Autodesk Fusion 360 part; units mm, degrees
(part 3 of 5)
  spline S639 degree 3 poles (-49.8546, -125.9974) (-49.939, -126.4512) (-49.939, -126.3246) (-49.9074, -125.2905) knots 0 0 0 0 1 1 1 1
  spline S640 degree 3 poles (-49.9074, -125.2905) (-49.8441, -123.6338) (-49.6436, -122.7158) (-49.3165, -122.4942) knots 0 0 0 0 1 1 1 1
  spline S641 degree 3 poles (-49.3165, -122.4942) (-48.926, -122.2515) (-48.1663, -121.5339) (-48.1663, -121.4179) knots 0 0 0 0 1 1 1 1
  spline S642 degree 3 poles (-48.1663, -121.4179) (-48.1663, -121.3545) (-48.409, -121.5339) (-48.7044, -121.7977) knots 0 0 0 0 1 1 1 1
  spline S643 degree 3 poles (-48.7044, -121.7977) (-49.1371, -122.1882) (-50.1923, -122.8107) (-50.4244, -122.8107) knots 0 0 0 0 1 1 1 1
  spline S644 degree 3 poles (-50.4244, -122.8107) (-50.4561, -122.8107) (-50.2345, -122.5575) (-49.9285, -122.2515) knots 0 0 0 0 1 1 1 1
  spline S645 degree 3 poles (-49.9285, -122.2515) (-49.633, -121.9349) (-49.327, -121.6184) (-49.2637, -121.5339) knots 0 0 0 0 1 1 1 1
  spline S646 degree 3 poles (-49.2637, -121.5339) (-49.2004, -121.4495) (-48.926, -121.2068) (-48.6622, -120.9852) knots 0 0 0 0 1 1 1 1
  spline S647 degree 3 poles (-48.6622, -120.9852) (-48.1979, -120.6054) (-47.4593, -119.6768) (-47.5543, -119.5818) knots 0 0 0 0 1 1 1 1
  spline S648 degree 3 poles (-47.5543, -119.5818) (-47.5859, -119.5607) (-47.8392, -119.8245) (-48.1241, -120.1727) knots 0 0 0 0 1 1 1 1
  spline S649 degree 3 poles (-48.1241, -120.1727) (-48.8944, -121.1013) (-49.7807, -121.7239) (-50.646, -121.9455) knots 0 0 0 0 1 1 1 1
  spline S650 degree 3 poles (-50.646, -121.9455) (-51.7012, -122.2093) (-51.6907, -122.2304) (-50.7093, -121.2596) knots 0 0 0 0 1 1 1 1
  spline S651 degree 3 poles (-50.7093, -121.2596) (-50.0129, -120.5631) (-49.6963, -120.1516) (-49.4431, -119.6346) knots 0 0 0 0 1 1 1 1
  spline S652 degree 3 poles (-49.4431, -119.6346) (-49.2637, -119.2441) (-49.116, -118.8959) (-49.116, -118.8537) knots 0 0 0 0 1 1 1 1
  spline S653 degree 3 poles (-49.116, -118.8537) (-49.116, -118.8115) (-49.2637, -118.9276) (-49.4536, -119.107) knots 0 0 0 0 1 1 1 1
  spline S654 degree 3 poles (-49.4536, -119.107) (-49.7491, -119.4024) (-50.7199, -119.8562) (-51.0364, -119.8562) knots 0 0 0 0 1 1 1 1
  spline S655 degree 3 poles (-51.0364, -119.8562) (-51.0998, -119.8562) (-50.9626, -119.6873) (-50.7304, -119.4868) knots 0 0 0 0 1 1 1 1
  spline S656 degree 3 poles (-50.7304, -119.4868) (-50.1606, -119.0014) (-49.3587, -117.9779) (-48.8311, -117.0599) knots 0 0 0 0 1 1 1 1
  spline S657 degree 3 poles (-48.8311, -117.0599) (-48.314, -116.163) (-47.5015, -113.8732) (-47.8075, -114.1792) knots 0 0 0 0 1 1 1 1
  spline S658 degree 3 poles (-47.8075, -114.1792) (-47.8392, -114.2214) (-48.0186, -114.6962) (-48.2085, -115.2449) knots 0 0 0 0 1 1 1 1
  spline S659 degree 3 poles (-48.2085, -115.2449) (-48.5145, -116.0996) (-49.1898, -117.5242) (-49.4325, -117.7774) knots 0 0 0 0 1 1 1 1
  spline S660 degree 3 poles (-49.4325, -117.7774) (-49.4642, -117.8196) (-49.3903, -117.5136) (-49.2531, -117.0915) knots 0 0 0 0 1 1 1 1
  spline S661 degree 3 poles (-49.2531, -117.0915) (-48.8944, -116.0047) (-48.8944, -116.0363) (-48.8944, -114.5801) knots 0 0 0 0 1 1 1 1
  spline S662 degree 3 poles (-48.8944, -114.5801) (-48.8838, -111.5412) (-49.8124, -108.5233) (-51.3213, -106.6872) knots 0 0 0 0 1 1 1 1
  spline S663 degree 3 poles (-51.3213, -106.6872) (-51.9334, -105.9591) (-51.8912, -106.1807) (-51.2791, -107.0038) knots 0 0 0 0 1 1 1 1
  spline S664 degree 3 poles (-52.8619, -111.5306) (-52.7142, -111.8261) (-52.6087, -112.0899) (-52.6192, -112.1004) knots 0 0 0 0 1 1 1 1
  spline S665 degree 3 poles (-52.6192, -112.1004) (-52.6403, -112.1215) (-52.8514, -112.1637) (-53.0941, -112.2059) knots 0 0 0 0 1 1 1 1
  line L120 (-53.0941, -112.2059) -> (-53.5373, -112.2798)
  line L121 (-53.5373, -112.2798) -> (-53.5267, -111.0769)
  line L122 (-53.5267, -111.0769) -> (-53.5162, -109.8845)
  line L123 (-53.5162, -109.8845) -> (-53.3262, -110.4332)
  spline S666 degree 3 poles (-53.3262, -110.4332) (-53.2313, -110.7392) (-53.0202, -111.2246) (-52.8619, -111.5306) knots 0 0 0 0 1 1 1 1
  spline S667 degree 3 poles (-59.8263, -110.8553) (-59.8263, -111.0769) (-59.7841, -111.499) (-59.7419, -111.805) knots 0 0 0 0 1 1 1 1
  line L124 (-59.7419, -111.805) -> (-59.668, -112.3537)
  line L125 (-59.668, -112.3537) -> (-60.0584, -112.2481)
  spline S668 degree 3 poles (-60.0584, -112.2481) (-60.7338, -112.0688) (-60.7549, -112.0582) (-60.6388, -111.9105) knots 0 0 0 0 1 1 1 1
  spline S669 degree 3 poles (-60.6388, -111.9105) (-60.5755, -111.8366) (-60.375, -111.4779) (-60.1956, -111.1191) knots 0 0 0 0 1 1 1 1
  spline S670 degree 3 poles (-60.1956, -111.1191) (-60.0162, -110.7603) (-59.8579, -110.4649) (-59.8474, -110.4649) knots 0 0 0 0 1 1 1 1
  spline S671 degree 3 poles (-59.8474, -110.4649) (-59.8368, -110.4649) (-59.8263, -110.6442) (-59.8263, -110.8553) knots 0 0 0 0 1 1 1 1
  spline S672 degree 3 poles (-50.1923, -114.0525) (-49.9812, -114.3691) (-49.6752, -114.8228) (-49.4958, -115.0444) knots 0 0 0 0 1 1 1 1
  spline S673 degree 3 poles (-49.4958, -115.0444) (-49.2215, -115.4032) (-49.2109, -115.4349) (-49.4114, -115.3293) knots 0 0 0 0 1 1 1 1
  spline S674 degree 3 poles (-49.4114, -115.3293) (-50.0551, -114.9811) (-52.4821, -112.2693) (-52.2288, -112.1848) knots 0 0 0 0 1 1 1 1
  spline S675 degree 3 poles (-52.2288, -112.1848) (-52.1655, -112.1637) (-51.9545, -112.0582) (-51.754, -111.9527) knots 0 0 0 0 1 1 1 1
  line L126 (-51.754, -111.9527) -> (-51.3847, -111.7522)
  line L127 (-51.3847, -111.7522) -> (-50.9731, -112.6175)
  spline S676 degree 3 poles (-50.9731, -112.6175) (-50.7515, -113.0818) (-50.4033, -113.736) (-50.1923, -114.0525) knots 0 0 0 0 1 1 1 1
  spline S677 degree 3 poles (-60.0268, -112.4381) (-59.6152, -112.5753) (-59.5836, -112.6175) (-59.4148, -113.2506) knots 0 0 0 0 1 1 1 1
  spline S678 degree 3 poles (-59.4148, -113.2506) (-59.1615, -114.1581) (-58.7816, -114.9495) (-58.3279, -115.5087) knots 0 0 0 0 1 1 1 1
  spline S679 degree 3 poles (-58.3279, -115.5087) (-57.8953, -116.0363) (-57.7897, -116.0258) (-58.0219, -115.4982) knots 0 0 0 0 1 1 1 1
  spline S680 degree 3 poles (-58.0219, -115.4982) (-58.2224, -115.0022) (-58.5495, -113.5249) (-58.4651, -113.4511) knots 0 0 0 0 1 1 1 1
  spline S681 degree 3 poles (-58.4651, -113.4511) (-58.4334, -113.4089) (-58.4018, -113.4511) (-58.4018, -113.5355) knots 0 0 0 0 1 1 1 1
  spline S682 degree 3 poles (-58.4018, -113.5355) (-58.4018, -113.8626) (-57.737, -115.0022) (-57.0722, -115.7936) knots 0 0 0 0 1 1 1 1
  spline S683 degree 3 poles (-57.0722, -115.7936) (-56.5763, -116.3951) (-56.5235, -116.5428) (-56.4918, -117.292) knots 0 0 0 0 1 1 1 1
  spline S684 degree 3 poles (-56.4918, -117.292) (-56.4707, -117.598) (-56.4391, -117.8513) (-56.3969, -117.8513) knots 0 0 0 0 1 1 1 1
  spline S685 degree 3 poles (-56.3969, -117.8513) (-56.3019, -117.8513) (-55.9748, -116.7855) (-55.9748, -116.469) knots 0 0 0 0 1 1 1 1
  spline S686 degree 3 poles (-55.9748, -116.469) (-55.9642, -116.2263) (-55.9537, -116.2368) (-55.7849, -116.5534) knots 0 0 0 0 1 1 1 1
  spline S687 degree 3 poles (-55.7849, -116.5534) (-55.5422, -117.0071) (-54.2865, -118.5899) (-54.1704, -118.5899) knots 0 0 0 0 1 1 1 1
  spline S688 degree 3 poles (-54.1704, -118.5899) (-54.1176, -118.5899) (-54.0649, -118.5055) (-54.0543, -118.4) knots 0 0 0 0 1 1 1 1
  spline S689 degree 3 poles (-54.0543, -118.4) (-54.0438, -118.305) (-54.0332, -118.1467) (-54.0121, -118.0623) knots 0 0 0 0 1 1 1 1
  spline S690 degree 3 poles (-54.0121, -118.0623) (-54.0016, -117.9779) (-53.991, -117.6824) (-53.9805, -117.3975) knots 0 0 0 0 1 1 1 1
  spline S691 degree 3 poles (-53.9805, -117.3975) (-53.9699, -116.9649) (-53.9382, -116.9016) (-53.7483, -116.9016) knots 0 0 0 0 1 1 1 1
  spline S692 degree 3 poles (-53.7483, -116.9016) (-53.5584, -116.9016) (-53.5267, -116.9544) (-53.5689, -117.2076) knots 0 0 0 0 1 1 1 1
  spline S693 degree 3 poles (-53.5689, -117.2076) (-53.6111, -117.482) (-53.5795, -117.5031) (-53.2946, -117.5031) knots 0 0 0 0 1 1 1 1
  spline S694 degree 3 poles (-53.2946, -117.5031) (-53.1152, -117.5031) (-53.0519, -117.482) (-53.1468, -117.4609) knots 0 0 0 0 1 1 1 1
  spline S695 degree 3 poles (-53.1468, -117.4609) (-53.2735, -117.4292) (-53.3368, -117.3131) (-53.3368, -117.1232) knots 0 0 0 0 1 1 1 1
  spline S696 degree 3 poles (-53.3368, -117.1232) (-53.3368, -116.8699) (-53.284, -116.8066) (-53.0097, -116.7539) knots 0 0 0 0 1 1 1 1
  spline S697 degree 3 poles (-53.0097, -116.7539) (-52.1972, -116.5956) (-51.8173, -116.7644) (-51.9334, -117.2287) knots 0 0 0 0 1 1 1 1
  spline S698 degree 3 poles (-51.9334, -117.2287) (-52.0072, -117.5136) (-52.5559, -117.5031) (-52.6509, -117.2182) knots 0 0 0 0 1 1 1 1
  spline S699 degree 3 poles (-52.6509, -117.2182) (-52.6826, -117.1021) (-52.6826, -116.9649) (-52.6509, -116.9016) knots 0 0 0 0 1 1 1 1
  spline S700 degree 3 poles (-52.6509, -116.9016) (-52.6192, -116.8488) (-52.6403, -116.7961) (-52.6931, -116.7961) knots 0 0 0 0 1 1 1 1
  spline S701 degree 3 poles (-52.6931, -116.7961) (-52.7564, -116.7961) (-52.8092, -116.9438) (-52.8092, -117.1126) knots 0 0 0 0 1 1 1 1
  spline S702 degree 3 poles (-52.8092, -117.1126) (-52.8092, -117.5031) (-52.6298, -117.5875) (-51.5957, -117.6824) knots 0 0 0 0 1 1 1 1
  line L128 (-51.5957, -117.6824) -> (-50.8571, -117.7563)
  line L129 (-50.8571, -117.7563) -> (-50.6566, -117.387)
  spline S703 degree 3 poles (-50.6566, -117.387) (-50.551, -117.1865) (-50.4877, -116.9438) (-50.5194, -116.8594) knots 0 0 0 0 1 1 1 1
  spline S704 degree 3 poles (-50.5194, -116.8594) (-50.5721, -116.7222) (-50.4983, -116.6906) (-50.0762, -116.6906) knots 0 0 0 0 1 1 1 1
  spline S705 degree 3 poles (-50.0762, -116.6906) (-49.8019, -116.6906) (-49.5486, -116.7222) (-49.5064, -116.7539) knots 0 0 0 0 1 1 1 1
  spline S706 degree 3 poles (-49.5064, -116.7539) (-49.4114, -116.8488) (-49.8652, -117.4292) (-50.034, -117.4292) knots 0 0 0 0 1 1 1 1
  spline S707 degree 3 poles (-50.034, -117.4292) (-50.1079, -117.4292) (-50.1712, -117.4714) (-50.1712, -117.5347) knots 0 0 0 0 1 1 1 1
  spline S708 degree 3 poles (-50.1712, -117.5347) (-50.1712, -117.5875) (-50.0445, -117.6402) (-49.8968, -117.6402) knots 0 0 0 0 1 1 1 1
  spline S709 degree 3 poles (-49.8968, -117.6402) (-49.7385, -117.6402) (-49.6541, -117.598) (-49.6963, -117.5347) knots 0 0 0 0 1 1 1 1
  spline S710 degree 3 poles (-49.6963, -117.5347) (-49.7385, -117.4714) (-49.7069, -117.3553) (-49.6436, -117.2709) knots 0 0 0 0 1 1 1 1
  spline S711 degree 3 poles (-49.6436, -117.2709) (-49.3692, -116.9332) (-49.3587, -117.1443) (-49.6119, -117.7458) knots 0 0 0 0 1 1 1 1
  spline S712 degree 3 poles (-49.6119, -117.7458) (-49.9074, -118.4105) (-50.7937, -119.4868) (-51.2686, -119.7401) knots 0 0 0 0 1 1 1 1
  spline S713 degree 3 poles (-51.2686, -119.7401) (-51.4163, -119.8245) (-51.5429, -119.9406) (-51.5429, -119.9933) knots 0 0 0 0 1 1 1 1
  spline S714 degree 3 poles (-51.5429, -119.9933) (-51.5429, -120.1727) (-50.6671, -119.9722) (-50.034, -119.6557) knots 0 0 0 0 1 1 1 1
  spline S715 degree 3 poles (-50.034, -119.6557) (-49.7069, -119.4763) (-49.4642, -119.4024) (-49.5064, -119.4657) knots 0 0 0 0 1 1 1 1
  spline S716 degree 3 poles (-49.5064, -119.4657) (-50.0657, -120.426) (-50.952, -121.4179) (-51.8067, -122.0404) knots 0 0 0 0 1 1 1 1
  line L130 (-51.8067, -122.0404) -> (-52.1233, -122.2726)
  line L131 (-52.1233, -122.2726) -> (-51.6485, -122.2726)
  spline S717 degree 3 poles (-51.6485, -122.2726) (-51.3847, -122.2726) (-50.9837, -122.2093) (-50.7515, -122.1248) knots 0 0 0 0 1 1 1 1
  spline S718 degree 3 poles (-50.7515, -122.1248) (-50.1712, -121.9138) (-50.1712, -121.9244) (-50.7304, -122.2831) knots 0 0 0 0 1 1 1 1
  spline S719 degree 3 poles (-50.7304, -122.2831) (-51.0048, -122.452) (-51.2791, -122.5997) (-51.3319, -122.5997) knots 0 0 0 0 1 1 1 1
  spline S720 degree 3 poles (-51.3319, -122.5997) (-51.3741, -122.5997) (-51.4374, -122.6419) (-51.4585, -122.6841) knots 0 0 0 0 1 1 1 1
  spline S721 degree 3 poles (-51.4585, -122.6841) (-51.5007, -122.8107) (-52.978, -123.37) (-53.9699, -123.6443) knots 0 0 0 0 1 1 1 1
  spline S722 degree 3 poles (-53.9699, -123.6443) (-55.4999, -124.0664) (-57.3571, -124.0348) (-59.2881, -123.5388) knots 0 0 0 0 1 1 1 1
  spline S723 degree 3 poles (-59.2881, -123.5388) (-60.4383, -123.2434) (-61.8945, -122.6419) (-62.1161, -122.357) knots 0 0 0 0 1 1 1 1
  spline S724 degree 3 poles (-62.1161, -122.357) (-62.306, -122.1248) (-62.9391, -121.0591) (-62.9391, -120.9747) knots 0 0 0 0 1 1 1 1
  spline S725 degree 3 poles (-62.9391, -120.9747) (-62.9391, -120.9536) (-62.7175, -121.038) (-62.4326, -121.1752) knots 0 0 0 0 1 1 1 1
  spline S726 degree 3 poles (-62.4326, -121.1752) (-61.7573, -121.5023) (-61.1875, -121.65) (-60.586, -121.65) knots 0 0 0 0 1 1 1 1
  spline S727 degree 3 poles (-60.586, -121.65) (-60.0162, -121.65) (-59.9529, -121.555) (-60.3961, -121.3545) knots 0 0 0 0 1 1 1 1
  spline S728 degree 3 poles (-60.3961, -121.3545) (-60.9026, -121.133) (-61.9367, -120.0566) (-62.1794, -119.5079) knots 0 0 0 0 1 1 1 1
  spline S729 degree 3 poles (-62.1794, -119.5079) (-62.306, -119.2336) (-62.4537, -118.7165) (-62.517, -118.3472) knots 0 0 0 0 1 1 1 1
  spline S730 degree 3 poles (-62.517, -118.3472) (-62.5804, -117.9885) (-62.6542, -117.6086) (-62.6753, -117.5136) knots 0 0 0 0 1 1 1 1
  spline S731 degree 3 poles (-62.6753, -117.5136) (-62.707, -117.3553) (-62.6331, -117.3659) (-62.2427, -117.598) knots 0 0 0 0 1 1 1 1
  spline S732 degree 3 poles (-62.2427, -117.598) (-61.7362, -117.8935) (-61.6201, -117.8513) (-62.0528, -117.5136) knots 0 0 0 0 1 1 1 1
  spline S733 degree 3 poles (-62.0528, -117.5136) (-62.3799, -117.2498) (-62.2849, -117.1337) (-61.7256, -117.0915) knots 0 0 0 0 1 1 1 1
  spline S734 degree 3 poles (-61.7256, -117.0915) (-61.3352, -117.0599) (-61.293, -117.0915) (-61.1875, -117.3764) knots 0 0 0 0 1 1 1 1
  spline S735 degree 3 poles (-61.1875, -117.3764) (-61.082, -117.6613) (-61.0292, -117.693) (-60.6599, -117.6719) knots 0 0 0 0 1 1 1 1
  spline S736 degree 3 poles (-60.6599, -117.6719) (-60.0901, -117.6508) (-60.0901, -117.6508) (-60.0901, -117.5453) knots 0 0 0 0 1 1 1 1
  spline S737 degree 3 poles (-60.0901, -117.5453) (-60.0901, -117.482) (-60.2484, -117.4714) (-60.4488, -117.5031) knots 0 0 0 0 1 1 1 1
  spline S738 degree 3 poles (-60.4488, -117.5031) (-60.7443, -117.5453) (-60.8287, -117.5136) (-60.9342, -117.3237) knots 0 0 0 0 1 1 1 1
  spline S739 degree 3 poles (-60.9342, -117.3237) (-60.9976, -117.197) (-61.0398, -117.081) (-61.0187, -117.0599) knots 0 0 0 0 1 1 1 1
  spline S740 degree 3 poles (-61.0187, -117.0599) (-60.9976, -117.0388) (-60.7443, -116.986) (-60.4488, -116.9544) knots 0 0 0 0 1 1 1 1
  line L132 (-60.4488, -116.9544) -> (-59.9107, -116.8805)
  line L133 (-59.9107, -116.8805) -> (-59.9529, -117.1865)
  spline S741 degree 3 poles (-59.9529, -117.1865) (-60.0162, -117.5875) (-59.7313, -117.8407) (-59.2776, -117.7774) knots 0 0 0 0 1 1 1 1
  spline S742 degree 3 poles (-59.2776, -117.7774) (-58.9083, -117.7141) (-58.7605, -117.4186) (-58.9399, -117.0915) knots 0 0 0 0 1 1 1 1
  spline S743 degree 3 poles (-58.9399, -117.0915) (-59.0243, -116.9227) (-59.0032, -116.9016) (-58.7394, -116.9016) knots 0 0 0 0 1 1 1 1
  spline S744 degree 3 poles (-58.7394, -116.9016) (-58.5073, -116.9016) (-58.4123, -116.9649) (-58.3595, -117.1337) knots 0 0 0 0 1 1 1 1
  spline S745 degree 3 poles (-58.3595, -117.1337) (-58.3279, -117.292) (-58.3595, -117.4186) (-58.4545, -117.4925) knots 0 0 0 0 1 1 1 1
  spline S746 degree 3 poles (-58.4545, -117.4925) (-58.6867, -117.6613) (-58.6445, -117.7669) (-58.4018, -117.6402) knots 0 0 0 0 1 1 1 1
  spline S747 degree 3 poles (-58.4018, -117.6402) (-58.2751, -117.5769) (-58.1907, -117.4186) (-58.1907, -117.2709) knots 0 0 0 0 1 1 1 1
  spline S748 degree 3 poles (-58.1907, -117.2709) (-58.1907, -117.0599) (-58.138, -117.0071) (-57.8953, -117.0071) knots 0 0 0 0 1 1 1 1
  spline S749 degree 3 poles (-57.8953, -117.0071) (-57.6315, -116.9966) (-57.6209, -116.986) (-57.8003, -116.8594) knots 0 0 0 0 1 1 1 1
  spline S750 degree 3 poles (-57.8003, -116.8594) (-57.9375, -116.7539) (-57.9586, -116.7011) (-57.853, -116.6589) knots 0 0 0 0 1 1 1 1
  spline S751 degree 3 poles (-57.853, -116.6589) (-57.7792, -116.6378) (-57.948, -116.5745) (-58.2329, -116.5323) knots 0 0 0 0 1 1 1 1
  spline S752 degree 3 poles (-58.2329, -116.5323) (-58.7394, -116.4479) (-60.2589, -116.5112) (-61.905, -116.6694) knots 0 0 0 0 1 1 1 1
  spline S753 degree 3 poles (-61.905, -116.6694) (-62.7175, -116.7433) (-62.7281, -116.7433) (-62.7281, -116.5006) knots 0 0 0 0 1 1 1 1
  spline S754 degree 3 poles (-62.7281, -116.5006) (-62.7281, -116.068) (-62.2955, -114.9706) (-61.7045, -113.8732) knots 0 0 0 0 1 1 1 1
  spline S755 degree 3 poles (-61.7045, -113.8732) (-61.3774, -113.2822) (-61.0714, -112.818) (-61.0292, -112.8496) knots 0 0 0 0 1 1 1 1
  spline S756 degree 3 poles (-61.0292, -112.8496) (-60.987, -112.8707) (-60.9131, -112.8391) (-60.8709, -112.7757) knots 0 0 0 0 1 1 1 1
  spline S757 degree 3 poles (-60.8709, -112.7757) (-60.8287, -112.6913) (-60.8393, -112.6808) (-60.9131, -112.723) knots 0 0 0 0 1 1 1 1
  spline S758 degree 3 poles (-60.9131, -112.723) (-61.0714, -112.818) (-61.0714, -112.7546) (-60.9131, -112.417) knots 0 0 0 0 1 1 1 1
  spline S759 degree 3 poles (-60.9131, -112.417) (-60.8287, -112.227) (-60.7338, -112.1637) (-60.6282, -112.2165) knots 0 0 0 0 1 1 1 1
  spline S760 degree 3 poles (-60.6282, -112.2165) (-60.5333, -112.2481) (-60.2589, -112.3537) (-60.0268, -112.4381) knots 0 0 0 0 1 1 1 1
  spline S761 degree 3 poles (-51.9861, -112.9762) (-51.3952, -113.7782) (-50.0762, -115.0761) (-49.4536, -115.4665) knots 0 0 0 0 1 1 1 1
  spline S762 degree 3 poles (-49.4536, -115.4665) (-49.1054, -115.6881) (-49.0421, -115.7725) (-49.0843, -115.9941) knots 0 0 0 0 1 1 1 1
  line L134 (-49.0843, -115.9941) -> (-49.1371, -116.2685)
  line L135 (-49.1371, -116.2685) -> (-50.8993, -116.2685)
  spline S763 degree 3 poles (-50.8993, -116.2685) (-51.87, -116.2685) (-52.9358, -116.3212) (-53.2735, -116.3845) knots 0 0 0 0 1 1 1 1
  spline S764 degree 3 poles (-53.2735, -116.3845) (-53.6111, -116.4479) (-53.9066, -116.4795) (-53.9171, -116.4584) knots 0 0 0 0 1 1 1 1
  spline S765 degree 3 poles (-53.9171, -116.4584) (-54.0332, -116.3423) (-53.9594, -114.5907) (-53.8011, -113.7149) knots 0 0 0 0 1 1 1 1
  line L136 (-53.8011, -113.7149) -> (-53.6111, -112.6913)
  line L137 (-53.6111, -112.6913) -> (-53.1574, -112.5647)
  spline S766 degree 3 poles (-53.1574, -112.5647) (-52.9041, -112.5014) (-52.672, -112.3959) (-52.6403, -112.3537) knots 0 0 0 0 1 1 1 1
  spline S767 degree 3 poles (-52.6403, -112.3537) (-52.5559, -112.2165) (-52.5559, -112.2059) (-51.9861, -112.9762) knots 0 0 0 0 1 1 1 1
  spline S768 degree 3 poles (-53.284, -112.4697) (-53.5795, -112.5964) (-53.6744, -112.5964) (-53.6006, -112.4697) knots 0 0 0 0 1 1 1 1
  spline S769 degree 3 poles (-53.6006, -112.4697) (-53.5689, -112.4064) (-53.4317, -112.3642) (-53.3051, -112.3748) knots 0 0 0 0 1 1 1 1
  spline S770 degree 3 poles (-53.3051, -112.3748) (-53.0835, -112.3748) (-53.0835, -112.3853) (-53.284, -112.4697) knots 0 0 0 0 1 1 1 1
  spline S771 degree 3 poles (-58.8766, -112.7863) (-58.7922, -112.7863) (-58.7183, -113.0079) (-58.6761, -113.4089) knots 0 0 0 0 1 1 1 1
  spline S772 degree 3 poles (-58.6761, -113.4089) (-58.6339, -113.7571) (-58.5178, -114.3586) (-58.4018, -114.7595) knots 0 0 0 0 1 1 1 1
  spline S773 degree 3 poles (-58.4018, -114.7595) (-58.2118, -115.4665) (-58.2118, -115.4665) (-58.4123, -115.2133) knots 0 0 0 0 1 1 1 1
  spline S774 degree 3 poles (-58.4123, -115.2133) (-58.6339, -114.9178) (-59.2143, -113.4827) (-59.3198, -112.9762) knots 0 0 0 0 1 1 1 1
  spline S775 degree 3 poles (-59.3198, -112.9762) (-59.3725, -112.6913) (-59.362, -112.6597) (-59.2037, -112.7124) knots 0 0 0 0 1 1 1 1
  spline S776 degree 3 poles (-59.2037, -112.7124) (-59.0982, -112.7546) (-58.961, -112.7863) (-58.8766, -112.7863) knots 0 0 0 0 1 1 1 1
  spline S777 degree 3 poles (-51.7962, -116.5323) (-51.7012, -116.6272) (-51.4374, -116.6906) (-51.1631, -116.6906) knots 0 0 0 0 1 1 1 1
  spline S778 degree 3 poles (-51.1631, -116.6906) (-50.6566, -116.6906) (-50.6249, -116.7328) (-50.8465, -117.2709) knots 0 0 0 0 1 1 1 1
  spline S779 degree 3 poles (-50.8465, -117.2709) (-51.0048, -117.6508) (-51.1314, -117.693) (-51.6168, -117.5558) knots 0 0 0 0 1 1 1 1
  spline S780 degree 3 poles (-51.6168, -117.5558) (-51.7856, -117.5031) (-51.8278, -117.4397) (-51.7645, -117.3342) knots 0 0 0 0 1 1 1 1
  spline S781 degree 3 poles (-51.7645, -117.3342) (-51.5324, -116.9649) (-51.9334, -116.4373) (-52.366, -116.5534) knots 0 0 0 0 1 1 1 1
  spline S782 degree 3 poles (-52.366, -116.5534) (-52.5454, -116.5956) (-52.6087, -116.5745) (-52.5559, -116.4901) knots 0 0 0 0 1 1 1 1
  spline S783 degree 3 poles (-52.5559, -116.4901) (-52.4504, -116.3212) (-51.9756, -116.3423) (-51.7962, -116.5323) knots 0 0 0 0 1 1 1 1
  spline S784 degree 3 poles (-59.7208, -116.6906) (-59.7524, -116.7433) (-59.8579, -116.7961) (-59.9424, -116.7961) knots 0 0 0 0 1 1 1 1
  spline S785 degree 3 poles (-59.9424, -116.7961) (-60.0268, -116.7961) (-60.0901, -116.7433) (-60.0901, -116.6906) knots 0 0 0 0 1 1 1 1
  spline S786 degree 3 poles (-60.0901, -116.6906) (-60.0901, -116.6272) (-59.9951, -116.585) (-59.8685, -116.585) knots 0 0 0 0 1 1 1 1
  spline S787 degree 3 poles (-59.8685, -116.585) (-59.7524, -116.585) (-59.6891, -116.6272) (-59.7208, -116.6906) knots 0 0 0 0 1 1 1 1
  spline S788 degree 3 poles (-53.7589, -116.6272) (-53.7589, -116.6589) (-53.8011, -116.7117) (-53.8644, -116.7433) knots 0 0 0 0 1 1 1 1
  spline S789 degree 3 poles (-53.8644, -116.7433) (-53.9171, -116.775) (-53.9699, -116.7539) (-53.9699, -116.7011) knots 0 0 0 0 1 1 1 1
  spline S790 degree 3 poles (-53.9699, -116.7011) (-53.9699, -116.6378) (-53.9171, -116.585) (-53.8644, -116.585) knots 0 0 0 0 1 1 1 1
  spline S791 degree 3 poles (-53.8644, -116.585) (-53.8011, -116.585) (-53.7589, -116.6061) (-53.7589, -116.6272) knots 0 0 0 0 1 1 1 1
  spline S792 degree 3 poles (-59.0982, -117.0704) (-58.9821, -117.3764) (-59.0349, -117.5453) (-59.267, -117.6297) knots 0 0 0 0 1 1 1 1
  spline S793 degree 3 poles (-59.267, -117.6297) (-59.5836, -117.7458) (-59.7735, -117.5875) (-59.7735, -117.2076) knots 0 0 0 0 1 1 1 1
  spline S794 degree 3 poles (-59.7735, -117.2076) (-59.7735, -116.9438) (-59.7313, -116.9016) (-59.4675, -116.9016) knots 0 0 0 0 1 1 1 1
  spline S795 degree 3 poles (-59.4675, -116.9016) (-59.2881, -116.9016) (-59.1404, -116.9649) (-59.0982, -117.0704) knots 0 0 0 0 1 1 1 1
  spline S796 degree 3 poles (-62.3377, -117.0704) (-62.3693, -117.1021) (-62.4643, -117.1126) (-62.5382, -117.081) knots 0 0 0 0 1 1 1 1
  spline S797 degree 3 poles (-62.5382, -117.081) (-62.6226, -117.0493) (-62.5909, -117.0177) (-62.4748, -117.0177) knots 0 0 0 0 1 1 1 1
  spline S798 degree 3 poles (-62.4748, -117.0177) (-62.3588, -117.0071) (-62.2955, -117.0388) (-62.3377, -117.0704) knots 0 0 0 0 1 1 1 1
  spline S799 degree 3 poles (-49.9074, -122.0826) (-50.1395, -122.3148) (-50.5299, -122.6208) (-50.7832, -122.7685) knots 0 0 0 0 1 1 1 1
  spline S800 degree 3 poles (-50.7832, -122.7685) (-51.0364, -122.9162) (-51.2264, -123.064) (-51.2053, -123.0851) knots 0 0 0 0 1 1 1 1
  spline S801 degree 3 poles (-51.2053, -123.0851) (-51.1525, -123.1273) (-50.2556, -122.8951) (-49.9179, -122.758) knots 0 0 0 0 1 1 1 1
  spline S802 degree 3 poles (-49.9179, -122.758) (-49.7596, -122.6841) (-49.7385, -122.7052) (-49.7807, -122.874) knots 0 0 0 0 1 1 1 1
  spline S803 degree 3 poles (-49.7807, -122.874) (-49.9285, -123.3489) (-50.0657, -124.5096) (-50.0657, -125.2799) knots 0 0 0 0 1 1 1 1
  line L138 (-50.0657, -125.2799) -> (-50.0657, -126.103)
  line L139 (-50.0657, -126.103) -> (-50.34, -126.0397)
  spline S804 degree 3 poles (-50.34, -126.0397) (-50.4983, -125.9974) (-50.7621, -125.9341) (-50.952, -125.9025) knots 0 0 0 0 1 1 1 1
  spline S805 degree 3 poles (-50.952, -125.9025) (-51.1314, -125.8708) (-51.3319, -125.797) (-51.4058, -125.7442) knots 0 0 0 0 1 1 1 1
  spline S806 degree 3 poles (-51.4058, -125.7442) (-51.5429, -125.6387) (-51.8173, -124.5096) (-51.9123, -123.6865) knots 0 0 0 0 1 1 1 1
  line L140 (-51.9123, -123.6865) -> (-51.965, -123.1484)
  line L141 (-51.965, -123.1484) -> (-51.4163, -122.874)
  spline S807 degree 3 poles (-51.4163, -122.874) (-51.1103, -122.7158) (-50.5721, -122.3886) (-50.2239, -122.1248) knots 0 0 0 0 1 1 1 1
  spline S808 degree 3 poles (-50.2239, -122.1248) (-49.8757, -121.861) (-49.5697, -121.65) (-49.5486, -121.65) knots 0 0 0 0 1 1 1 1
  spline S809 degree 3 poles (-49.5486, -121.65) (-49.5169, -121.65) (-49.6858, -121.8399) (-49.9074, -122.0826) knots 0 0 0 0 1 1 1 1
  spline S810 degree 3 poles (-52.0705, -123.5388) (-52.0705, -123.8659) (-51.8173, -125.1533) (-51.6907, -125.4909) knots 0 0 0 0 1 1 1 1
  spline S811 degree 3 poles (-51.6907, -125.4909) (-51.6274, -125.6598) (-51.6485, -125.6703) (-51.8278, -125.5754) knots 0 0 0 0 1 1 1 1
  spline S812 degree 3 poles (-51.8278, -125.5754) (-51.9439, -125.512) (-52.0705, -125.4804) (-52.1022, -125.512) knots 0 0 0 0 1 1 1 1
  spline S813 degree 3 poles (-52.1022, -125.512) (-52.1338, -125.5437) (-52.2499, -125.5226) (-52.3765, -125.4593) knots 0 0 0 0 1 1 1 1
  spline S814 degree 3 poles (-52.3765, -125.4593) (-52.6298, -125.3116) (-52.8092, -124.7418) (-52.8092, -124.0137) knots 0 0 0 0 1 1 1 1
  spline S815 degree 3 poles (-52.8092, -124.0137) (-52.8092, -123.5388) (-52.7775, -123.4755) (-52.5137, -123.37) knots 0 0 0 0 1 1 1 1
  spline S816 degree 3 poles (-52.5137, -123.37) (-52.0916, -123.2012) (-52.0705, -123.2012) (-52.0705, -123.5388) knots 0 0 0 0 1 1 1 1
  spline S817 degree 3 poles (-59.8263, -123.8448) (-59.7946, -124.0031) (-59.7735, -124.5518) (-59.7946, -125.0583) knots 0 0 0 0 1 1 1 1
  line L142 (-59.7946, -125.0583) -> (-59.8157, -125.9869)
  line L143 (-59.8157, -125.9869) -> (-60.1428, -126.1241)
  spline S818 degree 3 poles (-60.1428, -126.1241) (-60.3328, -126.2085) (-60.5755, -126.3035) (-60.7021, -126.3351) knots 0 0 0 0 1 1 1 1
  line L144 (-60.7021, -126.3351) -> (-60.9237, -126.409)
  line L145 (-60.9237, -126.409) -> (-60.7021, -125.9025)
  spline S819 degree 3 poles (-60.7021, -125.9025) (-60.3961, -125.206) (-60.1956, -124.4252) (-60.1956, -123.8976) knots 0 0 0 0 1 1 1 1
  spline S820 degree 3 poles (-60.1956, -123.8976) (-60.1956, -123.5494) (-60.1639, -123.465) (-60.0479, -123.5072) knots 0 0 0 0 1 1 1 1
  spline S821 degree 3 poles (-60.0479, -123.5072) (-59.9635, -123.5388) (-59.8685, -123.6971) (-59.8263, -123.8448) knots 0 0 0 0 1 1 1 1
  spline S822 degree 3 poles (-52.9358, -124.2247) (-52.9675, -124.8367) (-52.9886, -124.8895) (-53.1363, -124.7523) knots 0 0 0 0 1 1 1 1
  spline S823 degree 3 poles (-53.1363, -124.7523) (-53.2207, -124.6679) (-53.3579, -124.6046) (-53.4317, -124.6046) knots 0 0 0 0 1 1 1 1
  spline S824 degree 3 poles (-53.4317, -124.6046) (-53.6428, -124.6046) (-53.5373, -123.7182) (-53.3157, -123.676) knots 0 0 0 0 1 1 1 1
  spline S825 degree 3 poles (-53.3157, -123.676) (-53.1785, -123.6549) (-53.1257, -123.7393) (-53.0941, -124.0453) knots 0 0 0 0 1 1 1 1
  line L146 (-53.0941, -124.0453) -> (-53.0519, -124.4463)
  line L147 (-53.0519, -124.4463) -> (-53.0413, -123.9926)
  spline S826 degree 3 poles (-53.0413, -123.9926) (-53.0308, -123.7499) (-52.9991, -123.5494) (-52.9675, -123.5494) knots 0 0 0 0 1 1 1 1
  spline S827 degree 3 poles (-52.9675, -123.5494) (-52.9358, -123.5494) (-52.9253, -123.8554) (-52.9358, -124.2247) knots 0 0 0 0 1 1 1 1
  spline S828 degree 3 poles (-59.2037, -123.7604) (-59.056, -123.8132) (-58.7078, -123.887) (-58.4334, -123.9292) knots 0 0 0 0 1 1 1 1
  spline S829 degree 3 poles (-58.4334, -123.9292) (-57.6526, -124.0348) (-57.4521, -124.1403) (-57.4521, -124.4463) knots 0 0 0 0 1 1 1 1
  spline S830 degree 3 poles (-57.4521, -124.4463) (-57.4521, -124.594) (-57.4837, -124.7101) (-57.5259, -124.7101) knots 0 0 0 0 1 1 1 1
  spline S831 degree 3 poles (-57.5259, -124.7101) (-57.5787, -124.7101) (-57.8636, -124.9528) (-58.1696, -125.2377) knots 0 0 0 0 1 1 1 1
  spline S832 degree 3 poles (-58.1696, -125.2377) (-58.4756, -125.5332) (-58.7711, -125.7442) (-58.8238, -125.7125) knots 0 0 0 0 1 1 1 1
  spline S833 degree 3 poles (-58.8238, -125.7125) (-58.8766, -125.6809) (-59.0876, -125.7231) (-59.2881, -125.8075) knots 0 0 0 0 1 1 1 1
  line L148 (-59.2881, -125.8075) -> (-59.6574, -125.9658)
  line L149 (-59.6574, -125.9658) -> (-59.6574, -124.9106)
  spline S834 degree 3 poles (-59.6574, -124.9106) (-59.6574, -124.3302) (-59.6891, -123.8132) (-59.7208, -123.7604) knots 0 0 0 0 1 1 1 1
  spline S835 degree 3 poles (-59.7208, -123.7604) (-59.8052, -123.6232) (-59.5519, -123.6232) (-59.2037, -123.7604) knots 0 0 0 0 1 1 1 1
  spline S836 degree 3 poles (-53.685, -124.2247) (-53.685, -124.689) (-53.685, -124.689) (-54.1704, -124.8156) knots 0 0 0 0 1 1 1 1
  spline S837 degree 3 poles (-54.1704, -124.8156) (-54.8246, -124.9844) (-56.4602, -125.0372) (-56.9456, -124.9106) knots 0 0 0 0 1 1 1 1
  spline S838 degree 3 poles (-56.9456, -124.9106) (-57.2938, -124.8156) (-57.3466, -124.7629) (-57.3466, -124.4885) knots 0 0 0 0 1 1 1 1
  spline S839 degree 3 poles (-57.3466, -124.4885) (-57.3466, -124.3091) (-57.3043, -124.193) (-57.2516, -124.2247) knots 0 0 0 0 1 1 1 1
  spline S840 degree 3 poles (-57.2516, -124.2247) (-56.8823, -124.4568) (-55.8587, -124.3513) (-54.3392, -123.9292) knots 0 0 0 0 1 1 1 1
  spline S841 degree 3 poles (-54.3392, -123.9292) (-54.0438, -123.8554) (-53.78, -123.7815) (-53.7483, -123.771) knots 0 0 0 0 1 1 1 1
  spline S842 degree 3 poles (-53.7483, -123.771) (-53.7167, -123.771) (-53.685, -123.9715) (-53.685, -124.2247) knots 0 0 0 0 1 1 1 1
  line L150 (-53.0308, -125.0689) -> (-52.7986, -125.3116)
  line L151 (-52.7986, -125.3116) -> (-53.0413, -125.4698)
  spline S843 degree 3 poles (-53.0413, -125.4698) (-53.6006, -125.8392) (-54.0332, -125.9974) (-54.5397, -126.0397) knots 0 0 0 0 1 1 1 1
  spline S844 degree 3 poles (-54.5397, -126.0397) (-55.004, -126.0819) (-55.2045, -126.0291) (-56.0064, -125.6387) knots 0 0 0 0 1 1 1 1
  line L152 (-56.0064, -125.6387) -> (-56.9456, -125.1849)
  line L153 (-56.9456, -125.1849) -> (-55.7954, -125.1638)
  spline S845 degree 3 poles (-55.7954, -125.1638) (-55.1201, -125.1533) (-54.4658, -125.0794) (-54.1809, -124.995) knots 0 0 0 0 1 1 1 1
  spline S846 degree 3 poles (-54.1809, -124.995) (-53.5056, -124.7734) (-53.2946, -124.784) (-53.0308, -125.0689) knots 0 0 0 0 1 1 1 1
  spline S847 degree 3 poles (-55.2784, -126.0819) (-55.1939, -126.0819) (-55.1306, -126.1241) (-55.1306, -126.1874) knots 0 0 0 0 1 1 1 1
  spline S848 degree 3 poles (-55.1306, -126.1874) (-55.1306, -126.2507) (-55.4366, -126.2929) (-55.8482, -126.2929) knots 0 0 0 0 1 1 1 1
  spline S849 degree 3 poles (-55.8482, -126.2929) (-56.5974, -126.2929) (-57.5365, -126.0502) (-58.0324, -125.7231) knots 0 0 0 0 1 1 1 1
  line L154 (-58.0324, -125.7231) -> (-58.3173, -125.5332)
  line L155 (-58.3173, -125.5332) -> (-57.9691, -125.2482)
  line L156 (-57.9691, -125.2482) -> (-57.6209, -124.9528)
  line L157 (-57.6209, -124.9528) -> (-56.5235, -125.5226)
  spline S850 degree 3 poles (-56.5235, -125.5226) (-55.922, -125.8286) (-55.3628, -126.0819) (-55.2784, -126.0819) knots 0 0 0 0 1 1 1 1
  spline S851 degree 3 poles (-52.4926, -125.5543) (-52.3554, -125.6492) (-52.3871, -125.7125) (-52.6509, -125.9447) knots 0 0 0 0 1 1 1 1
  line L158 (-52.6509, -125.9447) -> (-52.9675, -126.219)
  line L159 (-52.9675, -126.219) -> (-52.9991, -125.9869)
  spline S852 degree 3 poles (-52.9991, -125.9869) (-53.0308, -125.7653) (-52.8619, -125.4487) (-52.7142, -125.4487) knots 0 0 0 0 1 1 1 1
  spline S853 degree 3 poles (-52.7142, -125.4487) (-52.6826, -125.4487) (-52.577, -125.5015) (-52.4926, -125.5543) knots 0 0 0 0 1 1 1 1
  spline S854 degree 3 poles (-58.2435, -125.7653) (-58.1591, -125.9025) (-57.6209, -126.1874) (-57.3149, -126.2612) knots 0 0 0 0 1 1 1 1
  spline S855 degree 3 poles (-57.3149, -126.2612) (-56.5868, -126.4301) (-56.2386, -126.4723) (-55.8376, -126.4512) knots 0 0 0 0 1 1 1 1
  spline S856 degree 3 poles (-55.8376, -126.4512) (-55.1834, -126.409) (-54.3814, -126.2823) (-54.086, -126.1768) knots 0 0 0 0 1 1 1 1
  spline S857 degree 3 poles (-54.086, -126.1768) (-53.7905, -126.0608) (-53.7905, -126.0502) (-53.7378, -126.4406) knots 0 0 0 0 1 1 1 1
  spline S858 degree 3 poles (-53.7378, -126.4406) (-53.7061, -126.715) (-53.7483, -126.7677) (-54.1282, -126.9049) knots 0 0 0 0 1 1 1 1
  spline S859 degree 3 poles (-54.1282, -126.9049) (-54.392, -126.9999) (-54.9618, -127.0632) (-55.6582, -127.0737) knots 0 0 0 0 1 1 1 1
  spline S860 degree 3 poles (-55.6582, -127.0737) (-56.6501, -127.0843) (-56.8295, -127.0526) (-57.3466, -126.8099) knots 0 0 0 0 1 1 1 1
  spline S861 degree 3 poles (-57.3466, -126.8099) (-58.1063, -126.4617) (-58.7816, -125.8708) (-58.5917, -125.7547) knots 0 0 0 0 1 1 1 1
  spline S862 degree 3 poles (-58.5917, -125.7547) (-58.4123, -125.6387) (-58.3173, -125.6387) (-58.2435, -125.7653) knots 0 0 0 0 1 1 1 1
  spline S863 degree 3 poles (-51.7751, -125.7547) (-51.659, -125.8181) (-51.7012, -125.9236) (-51.9545, -126.2085) knots 0 0 0 0 1 1 1 1
  line L160 (-51.9545, -126.2085) -> (-52.271, -126.5778)
  line L161 (-52.271, -126.5778) -> (-52.0283, -127.6225)
  spline S864 degree 3 poles (-52.0283, -127.6225) (-51.6379, -129.2158) (-51.6168, -129.4585) (-51.7962, -129.4585) knots 0 0 0 0 1 1 1 1
  spline S865 degree 3 poles (-51.7962, -129.4585) (-51.8806, -129.4585) (-52.0178, -129.4902) (-52.1127, -129.5218) knots 0 0 0 0 1 1 1 1
  spline S866 degree 3 poles (-52.1127, -129.5218) (-52.2394, -129.5746) (-52.2816, -129.5218) (-52.2816, -129.3213) knots 0 0 0 0 1 1 1 1
  spline S867 degree 3 poles (-52.2816, -129.3213) (-52.2816, -129.1736) (-52.3343, -128.9204) (-52.3871, -128.7621) knots 0 0 0 0 1 1 1 1
  line L162 (-52.3871, -128.7621) -> (-52.5032, -128.4772)
  line L163 (-52.5032, -128.4772) -> (-52.2183, -128.6671)
  line L164 (-52.2183, -128.6671) -> (-51.9334, -128.8465)
  line L165 (-51.9334, -128.8465) -> (-51.9967, -128.3928)
  spline S868 degree 3 poles (-51.9967, -128.3928) (-52.0283, -128.1395) (-52.1444, -127.8546) (-52.2499, -127.7702) knots 0 0 0 0 1 1 1 1
  spline S869 degree 3 poles (-52.2499, -127.7702) (-52.3554, -127.6752) (-52.4926, -127.5064) (-52.5665, -127.3798) knots 0 0 0 0 1 1 1 1
  spline S870 degree 3 poles (-52.5665, -127.3798) (-52.6615, -127.2004) (-52.6509, -127.1265) (-52.461, -126.9366) knots 0 0 0 0 1 1 1 1
  spline S871 degree 3 poles (-52.461, -126.9366) (-52.3343, -126.8205) (-52.2816, -126.715) (-52.3449, -126.715) knots 0 0 0 0 1 1 1 1
  spline S872 degree 3 poles (-52.3449, -126.715) (-52.4082, -126.715) (-52.5665, -126.8311) (-52.7037, -126.9788) knots 0 0 0 0 1 1 1 1
  spline S873 degree 3 poles (-52.7037, -126.9788) (-52.9253, -127.2109) (-52.9253, -127.2426) (-52.767, -127.3059) knots 0 0 0 0 1 1 1 1
  spline S874 degree 3 poles (-52.767, -127.3059) (-52.6509, -127.3481) (-52.5981, -127.4536) (-52.6298, -127.5697) knots 0 0 0 0 1 1 1 1
  spline S875 degree 3 poles (-52.6298, -127.5697) (-52.6615, -127.6858) (-52.6298, -127.7702) (-52.5454, -127.7702) knots 0 0 0 0 1 1 1 1
  spline S876 degree 3 poles (-52.5454, -127.7702) (-52.366, -127.7702) (-52.2077, -127.9707) (-52.1127, -128.34) knots 0 0 0 0 1 1 1 1
  line L166 (-52.1127, -128.34) -> (-52.0389, -128.6566)
  line L167 (-52.0389, -128.6566) -> (-52.366, -128.4139)
  spline S877 degree 3 poles (-52.366, -128.4139) (-52.5559, -128.2872) (-52.7037, -128.0867) (-52.7037, -127.9812) knots 0 0 0 0 1 1 1 1
  spline S878 degree 3 poles (-52.7037, -127.9812) (-52.7037, -127.8757) (-52.7775, -127.7702) (-52.8619, -127.7385) knots 0 0 0 0 1 1 1 1
  spline S879 degree 3 poles (-52.8619, -127.7385) (-52.9464, -127.6963) (-52.9886, -127.5802) (-52.9675, -127.4536) knots 0 0 0 0 1 1 1 1
  spline S880 degree 3 poles (-52.9675, -127.4536) (-52.9464, -127.327) (-52.9569, -127.2426) (-52.9991, -127.2637) knots 0 0 0 0 1 1 1 1
  spline S881 degree 3 poles (-52.9991, -127.2637) (-54.8352, -128.2239) (-56.3441, -128.3083) (-57.8214, -127.5275) knots 0 0 0 0 1 1 1 1
  spline S882 degree 3 poles (-57.8214, -127.5275) (-58.4018, -127.2215) (-59.457, -126.2929) (-59.457, -126.0924) knots 0 0 0 0 1 1 1 1
  spline S883 degree 3 poles (-59.457, -126.0924) (-59.457, -126.0502) (-59.3409, -125.9552) (-59.2037, -125.8919) knots 0 0 0 0 1 1 1 1
  spline S884 degree 3 poles (-59.2037, -125.8919) (-58.9716, -125.7864) (-58.8871, -125.8286) (-58.3595, -126.2929) knots 0 0 0 0 1 1 1 1
  spline S885 degree 3 poles (-58.3595, -126.2929) (-57.547, -126.9999) (-56.8295, -127.2531) (-55.616, -127.2531) knots 0 0 0 0 1 1 1 1
  spline S886 degree 3 poles (-55.616, -127.2531) (-54.392, -127.2531) (-53.7061, -126.9999) (-52.7986, -126.2401) knots 0 0 0 0 1 1 1 1
  spline S887 degree 3 poles (-52.7986, -126.2401) (-52.0916, -125.6492) (-52.0072, -125.607) (-51.7751, -125.7547) knots 0 0 0 0 1 1 1 1
  spline S888 degree 3 poles (-53.284, -126.4934) (-53.4317, -126.6411) (-53.4634, -126.6411) (-53.5478, -126.5039) knots 0 0 0 0 1 1 1 1
  spline S889 degree 3 poles (-53.5478, -126.5039) (-53.7167, -126.2296) (-53.6639, -125.9763) (-53.4106, -125.8814) knots 0 0 0 0 1 1 1 1
  spline S890 degree 3 poles (-53.4106, -125.8814) (-53.2102, -125.8075) (-53.1785, -125.8286) (-53.1468, -126.0608) knots 0 0 0 0 1 1 1 1
  spline S891 degree 3 poles (-53.1468, -126.0608) (-53.1257, -126.1979) (-53.1891, -126.3984) (-53.284, -126.4934) knots 0 0 0 0 1 1 1 1
  spline S892 degree 3 poles (-50.9837, -126.9577) (-50.8887, -127.4958) (-50.7199, -128.2872) (-50.6038, -128.7199) knots 0 0 0 0 1 1 1 1
  spline S893 degree 3 poles (-50.6038, -128.7199) (-50.4877, -129.1525) (-50.4033, -129.5113) (-50.4139, -129.5218) knots 0 0 0 0 1 1 1 1
  spline S894 degree 3 poles (-50.4139, -129.5218) (-50.4244, -129.5324) (-50.5299, -129.5007) (-50.6566, -129.4585) knots 0 0 0 0 1 1 1 1
  spline S895 degree 3 poles (-50.6566, -129.4585) (-50.836, -129.3846) (-50.8887, -129.2475) (-50.9415, -128.7937) knots 0 0 0 0 1 1 1 1
  spline S896 degree 3 poles (-50.9415, -128.7937) (-50.9837, -128.4772) (-51.0786, -128.034) (-51.1631, -127.7913) knots 0 0 0 0 1 1 1 1
  spline S897 degree 3 poles (-51.1631, -127.7913) (-51.2475, -127.5591) (-51.353, -127.021) (-51.3952, -126.6095) knots 0 0 0 0 1 1 1 1
  spline S898 degree 3 poles (-51.3952, -126.6095) (-51.4585, -125.9763) (-51.4374, -125.8708) (-51.3108, -125.9236) knots 0 0 0 0 1 1 1 1
  spline S899 degree 3 poles (-51.3108, -125.9236) (-51.2053, -125.9658) (-51.0998, -126.3246) (-50.9837, -126.9577) knots 0 0 0 0 1 1 1 1
  spline S900 degree 3 poles (-50.5405, -126.1874) (-50.5088, -126.2401) (-50.4033, -126.7044) (-50.3189, -127.2109) knots 0 0 0 0 1 1 1 1
  spline S901 degree 3 poles (-50.3189, -127.2109) (-50.1395, -128.2239) (-50.1184, -128.3505) (-49.9496, -129.659) knots 0 0 0 0 1 1 1 1
  spline S902 degree 3 poles (-49.9496, -129.659) (-49.8335, -130.4821) (-49.5592, -131.4739) (-49.4009, -131.6428) knots 0 0 0 0 1 1 1 1
  spline S903 degree 3 poles (-49.4009, -131.6428) (-49.2954, -131.7483) (-49.3165, -132.7191) (-49.4325, -133.4261) knots 0 0 0 0 1 1 1 1
  spline S904 degree 3 poles (-49.4325, -133.4261) (-49.6014, -134.3758) (-49.8335, -134.9139) (-50.0868, -134.9878) knots 0 0 0 0 1 1 1 1
  spline S905 degree 3 poles (-50.0868, -134.9878) (-50.2134, -135.0194) (-50.3295, -135.03) (-50.34, -135.0194) knots 0 0 0 0 1 1 1 1
  spline S906 degree 3 poles (-50.34, -135.0194) (-50.3611, -135.0089) (-50.2767, -134.724) (-50.1606, -134.3758) knots 0 0 0 0 1 1 1 1
  spline S907 degree 3 poles (-50.1606, -134.3758) (-49.8968, -133.6055) (-49.8124, -132.2653) (-49.9601, -131.3051) knots 0 0 0 0 1 1 1 1
  spline S908 degree 3 poles (-49.9601, -131.3051) (-50.1923, -129.9122) (-50.4983, -128.3505) (-50.646, -127.9285) knots 0 0 0 0 1 1 1 1
  spline S909 degree 3 poles (-50.646, -127.9285) (-50.7304, -127.6963) (-50.8254, -127.2637) (-50.8571, -126.9788) knots 0 0 0 0 1 1 1 1
  spline S910 degree 3 poles (-50.8571, -126.9788) (-50.8887, -126.6833) (-50.9415, -126.3668) (-50.9731, -126.2612) knots 0 0 0 0 1 1 1 1
  spline S911 degree 3 poles (-50.9731, -126.2612) (-51.0153, -126.1346) (-50.9731, -126.0819) (-50.8148, -126.0819) knots 0 0 0 0 1 1 1 1
  spline S912 degree 3 poles (-50.8148, -126.0819) (-50.6988, -126.0819) (-50.5721, -126.1241) (-50.5405, -126.1874) knots 0 0 0 0 1 1 1 1
  spline S913 degree 3 poles (-59.0982, -126.7361) (-57.9797, -127.8863) (-56.1225, -128.4877) (-54.8457, -128.1184) knots 0 0 0 0 1 1 1 1
  spline S914 degree 3 poles (-54.8457, -128.1184) (-54.4447, -128.0023) (-54.4025, -128.0129) (-54.3287, -128.2239) knots 0 0 0 0 1 1 1 1
  spline S915 degree 3 poles (-54.3287, -128.2239) (-54.2865, -128.3505) (-54.2443, -128.5616) (-54.2337, -128.6777) knots 0 0 0 0 1 1 1 1
  spline S916 degree 3 poles (-54.2337, -128.6777) (-54.2126, -128.9626) (-53.6639, -129.6907) (-53.5373, -129.6062) knots 0 0 0 0 1 1 1 1
  spline S917 degree 3 poles (-53.5373, -129.6062) (-53.379, -129.5113) (-53.4317, -128.6566) (-53.6006, -128.5088) knots 0 0 0 0 1 1 1 1
  spline S918 degree 3 poles (-53.6006, -128.5088) (-53.685, -128.435) (-53.7272, -128.34) (-53.6956, -128.2767) knots 0 0 0 0 1 1 1 1
  spline S919 degree 3 poles (-53.6956, -128.2767) (-53.6639, -128.2239) (-53.6956, -128.1078) (-53.7694, -128.0234) knots 0 0 0 0 1 1 1 1
  spline S920 degree 3 poles (-53.7694, -128.0234) (-53.8749, -127.8863) (-53.8749, -127.844) (-53.7483, -127.7702) knots 0 0 0 0 1 1 1 1
  spline S921 degree 3 poles (-53.7483, -127.7702) (-53.5478, -127.6436) (-53.4001, -127.939) (-53.1785, -128.9731) knots 0 0 0 0 1 1 1 1
  spline S922 degree 3 poles (-53.1785, -128.9731) (-52.9569, -129.965) (-52.8725, -129.8489) (-54.4342, -130.6614) knots 0 0 0 0 1 1 1 1
  line L168 (-54.4342, -130.6614) -> (-55.4366, -131.1679)
  line L169 (-55.4366, -131.1679) -> (-56.3652, -130.6403)
  spline S923 degree 3 poles (-56.3652, -130.6403) (-57.2832, -130.1127) (-58.1907, -129.6801) (-58.5178, -129.6168) knots 0 0 0 0 1 1 1 1
  spline S924 degree 3 poles (-58.5178, -129.6168) (-58.6128, -129.5957) (-58.866, -129.5218) (-59.0982, -129.4585) knots 0 0 0 0 1 1 1 1
  spline S925 degree 3 poles (-59.0982, -129.4585) (-59.457, -129.353) (-59.5836, -129.3635) (-60.0584, -129.5535) knots 0 0 0 0 1 1 1 1
  spline S926 degree 3 poles (-60.0584, -129.5535) (-60.3644, -129.6695) (-60.6282, -129.7329) (-60.6493, -129.6907) knots 0 0 0 0 1 1 1 1
  spline S927 degree 3 poles (-60.6493, -129.6907) (-60.6704, -129.6484) (-60.7021, -129.3319) (-60.7126, -128.9942) knots 0 0 0 0 1 1 1 1
  spline S928 degree 3 poles (-60.7126, -128.9942) (-60.7232, -128.646) (-60.7654, -128.3189) (-60.7971, -128.2661) knots 0 0 0 0 1 1 1 1
  spline S929 degree 3 poles (-60.7971, -128.2661) (-60.9026, -128.0973) (-60.2695, -126.3035) (-60.0901, -126.2612) knots 0 0 0 0 1 1 1 1
  spline S930 degree 3 poles (-60.0901, -126.2612) (-59.7313, -126.1557) (-59.6258, -126.2085) (-59.0982, -126.7361) knots 0 0 0 0 1 1 1 1
  spline S931 degree 3 poles (-50.0973, -127.0421) (-50.0762, -127.9496) (-50.129, -127.9074) (-50.2556, -126.8944) knots 0 0 0 0 1 1 1 1
  spline S932 degree 3 poles (-50.2556, -126.8944) (-50.3189, -126.3879) (-50.3083, -126.1979) (-50.2345, -126.219) knots 0 0 0 0 1 1 1 1
  spline S933 degree 3 poles (-50.2345, -126.219) (-50.1712, -126.2401) (-50.1079, -126.5884) (-50.0973, -127.0421) knots 0 0 0 0 1 1 1 1
  spline S934 degree 3 poles (-60.6493, -127.0949) (-60.8393, -127.6752) (-60.892, -127.7491) (-60.9448, -127.5486) knots 0 0 0 0 1 1 1 1
  spline S935 degree 3 poles (-60.9448, -127.5486) (-61.082, -127.0632) (-61.0503, -126.62) (-60.8498, -126.5145) knots 0 0 0 0 1 1 1 1
  spline S936 degree 3 poles (-60.8498, -126.5145) (-60.4594, -126.2823) (-60.4172, -126.3879) (-60.6493, -127.0949) knots 0 0 0 0 1 1 1 1
  spline S937 degree 3 poles (-53.8538, -128.0445) (-53.7483, -128.1817) (-53.7483, -128.2239) (-53.8749, -128.3083) knots 0 0 0 0 1 1 1 1
  spline S938 degree 3 poles (-53.8749, -128.3083) (-54.0649, -128.435) (-54.1493, -128.4244) (-54.2337, -128.2978) knots 0 0 0 0 1 1 1 1
  spline S939 degree 3 poles (-54.2337, -128.2978) (-54.3181, -128.1606) (-54.2232, -127.8757) (-54.0965, -127.8757) knots 0 0 0 0 1 1 1 1
  spline S940 degree 3 poles (-54.0965, -127.8757) (-54.0438, -127.8757) (-53.9382, -127.9496) (-53.8538, -128.0445) knots 0 0 0 0 1 1 1 1
  spline S941 degree 3 poles (-53.5689, -129.0997) (-53.59, -129.3846) (-53.6217, -129.4269) (-53.7272, -129.3319) knots 0 0 0 0 1 1 1 1
  spline S942 degree 3 poles (-53.7272, -129.3319) (-53.8116, -129.2686) (-53.8538, -129.1631) (-53.8327, -129.0997) knots 0 0 0 0 1 1 1 1
  spline S943 degree 3 poles (-53.8327, -129.0997) (-53.8116, -129.0364) (-53.8327, -128.8887) (-53.8855, -128.7726) knots 0 0 0 0 1 1 1 1
  spline S944 degree 3 poles (-53.8855, -128.7726) (-53.9699, -128.5827) (-53.9699, -128.5827) (-53.9277, -128.8043) knots 0 0 0 0 1 1 1 1
  spline S945 degree 3 poles (-53.9277, -128.8043) (-53.9066, -128.9309) (-53.9277, -129.0153) (-53.9805, -128.9731) knots 0 0 0 0 1 1 1 1
  spline S946 degree 3 poles (-53.9805, -128.9731) (-54.086, -128.9098) (-54.1071, -128.5721) (-54.0016, -128.4772) knots 0 0 0 0 1 1 1 1
  spline S947 degree 3 poles (-54.0016, -128.4772) (-53.8538, -128.3189) (-53.5478, -128.7621) (-53.5689, -129.0997) knots 0 0 0 0 1 1 1 1
  spline S948 degree 3 poles (-42.5843, -129.4585) (-42.5843, -129.4902) (-42.6476, -129.6062) (-42.732, -129.7118) knots 0 0 0 0 1 1 1 1
  spline S949 degree 3 poles (-42.732, -129.7118) (-42.9219, -129.965) (-43.133, -129.8173) (-43.3862, -129.258) knots 0 0 0 0 1 1 1 1
  spline S950 degree 3 poles (-43.3862, -129.258) (-43.4812, -129.047) (-43.5762, -128.8359) (-43.6078, -128.7937) knots 0 0 0 0 1 1 1 1
  spline S951 degree 3 poles (-43.6078, -128.7937) (-43.6289, -128.741) (-43.4073, -128.857) (-43.1224, -129.0575) knots 0 0 0 0 1 1 1 1
  spline S952 degree 3 poles (-43.1224, -129.0575) (-42.827, -129.2475) (-42.5843, -129.4269) (-42.5843, -129.4585) knots 0 0 0 0 1 1 1 1
  spline S953 degree 3 poles (-46.0559, -129.2686) (-46.0559, -129.4057) (-46.2986, -129.3213) (-46.3513, -129.1631) knots 0 0 0 0 1 1 1 1
  spline S954 degree 3 poles (-46.3513, -129.1631) (-46.3724, -129.0892) (-46.3302, -129.0575) (-46.2247, -129.0997) knots 0 0 0 0 1 1 1 1
  spline S955 degree 3 poles (-46.2247, -129.0997) (-46.1297, -129.1314) (-46.0559, -129.2158) (-46.0559, -129.2686) knots 0 0 0 0 1 1 1 1
  spline S956 degree 3 poles (-45.1062, -129.5007) (-45.1062, -129.5218) (-45.1801, -129.564) (-45.2645, -129.6062) knots 0 0 0 0 1 1 1 1
  spline S957 degree 3 poles (-45.2645, -129.6062) (-45.3489, -129.6379) (-45.4228, -129.6168) (-45.4228, -129.564) knots 0 0 0 0 1 1 1 1
  spline S958 degree 3 poles (-45.4228, -129.564) (-45.4228, -129.5007) (-45.3489, -129.4585) (-45.2645, -129.4585) knots 0 0 0 0 1 1 1 1
  spline S959 degree 3 poles (-45.2645, -129.4585) (-45.1801, -129.4585) (-45.1062, -129.4796) (-45.1062, -129.5007) knots 0 0 0 0 1 1 1 1
  spline S960 degree 3 poles (-51.5007, -130.8514) (-51.5007, -131.3051) (-51.448, -131.6744) (-51.4058, -131.6744) knots 0 0 0 0 1 1 1 1
  spline S961 degree 3 poles (-51.4058, -131.6744) (-51.3213, -131.6744) (-51.3847, -132.8141) (-51.5007, -133.5949) knots 0 0 0 0 1 1 1 1
  spline S962 degree 3 poles (-51.5007, -133.5949) (-51.5535, -133.9326) (-51.6062, -133.9959) (-51.8173, -133.9959) knots 0 0 0 0 1 1 1 1
  spline S963 degree 3 poles (-51.8173, -133.9959) (-51.9545, -133.9959) (-52.0705, -133.9853) (-52.0705, -133.9642) knots 0 0 0 0 1 1 1 1
  spline S964 degree 3 poles (-52.0705, -133.9642) (-52.0705, -133.9537) (-52.0178, -133.7743) (-51.965, -133.5738) knots 0 0 0 0 1 1 1 1
  spline S965 degree 3 poles (-51.965, -133.5738) (-51.8595, -133.2045) (-51.8173, -131.073) (-51.9017, -130.672) knots 0 0 0 0 1 1 1 1
  spline S966 degree 3 poles (-51.9017, -130.672) (-51.9334, -130.5559) (-51.9967, -130.3027) (-52.06, -130.1127) knots 0 0 0 0 1 1 1 1
  spline S967 degree 3 poles (-52.06, -130.1127) (-52.155, -129.7962) (-52.1444, -129.754) (-51.9334, -129.6801) knots 0 0 0 0 1 1 1 1
  spline S968 degree 3 poles (-51.9334, -129.6801) (-51.6168, -129.564) (-51.5218, -129.8278) (-51.5007, -130.8514) knots 0 0 0 0 1 1 1 1
  spline S969 degree 3 poles (-50.2767, -130.2816) (-50.2134, -130.6192) (-50.129, -131.4528) (-50.0973, -132.1598) knots 0 0 0 0 1 1 1 1
  spline S970 degree 3 poles (-50.0973, -132.1598) (-50.034, -133.521) (-50.1184, -133.8904) (-50.4877, -133.8904) knots 0 0 0 0 1 1 1 1
  spline S971 degree 3 poles (-50.4877, -133.8904) (-50.6671, -133.8904) (-50.6777, -133.8376) (-50.6144, -133.5421) knots 0 0 0 0 1 1 1 1
  spline S972 degree 3 poles (-50.6144, -133.5421) (-50.4983, -133.0356) (-50.5299, -130.8619) (-50.6566, -130.1866) knots 0 0 0 0 1 1 1 1
  spline S973 degree 3 poles (-50.6566, -130.1866) (-50.7621, -129.6484) (-50.7515, -129.5957) (-50.5827, -129.6379) knots 0 0 0 0 1 1 1 1
  spline S974 degree 3 poles (-50.5827, -129.6379) (-50.4666, -129.6695) (-50.3611, -129.8806) (-50.2767, -130.2816) knots 0 0 0 0 1 1 1 1
  spline S975 degree 3 poles (-60.1639, -130.1655) (-60.2484, -130.4504) (-60.375, -131.1468) (-60.4488, -131.7166) knots 0 0 0 0 1 1 1 1
  spline S976 degree 3 poles (-60.4488, -131.7166) (-60.5649, -132.7613) (-60.5649, -132.7718) (-60.7549, -132.4869) knots 0 0 0 0 1 1 1 1
  spline S977 degree 3 poles (-60.7549, -132.4869) (-60.9237, -132.2337) (-60.9237, -132.1493) (-60.776, -131.4634) knots 0 0 0 0 1 1 1 1
  spline S978 degree 3 poles (-60.776, -131.4634) (-60.6915, -131.0519) (-60.6177, -130.5454) (-60.6177, -130.3554) knots 0 0 0 0 1 1 1 1